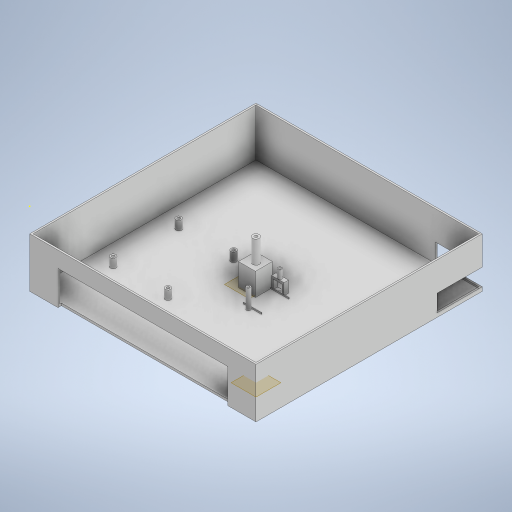
# Autodesk Inventor part: Box
Saved by Autodesk Inventor 2024 (Build 280153000, 153)
## iProperties
Created: 2023-12-20
Part Number: Box
Material: Generic
Document SubType Name: Modeling
Designer: 96279
Density: 1 g/cm^3
Appearance: Default
Author: 96279
Autodesk Inventor part; units mm, degrees
ref_plane "YZ Plane" through (0, 0, 0) normal (1, 0, 0) x (0, 1, 0)
ref_plane "XZ Plane" through (0, 0, 0) normal (0, 1, 0) x (-1, 0, 0)
ref_plane "XY Plane" through (0, 0, 0) normal (0, 0, 1) x (1, 0, 0)
sketch "Sketch1" plane through (0, 0, 0) normal (0, 1, 0) x (-1, 0, 0)
  line L0 (0, 0) -> (200, 0)
  line L1 (200, 0) -> (200, -200)
  line L2 (200, -200) -> (0, -200)
  line L3 (0, -200) -> (0, 0)
  line L4 (198, -198) -> (198, -2)
  line L5 (198, -2) -> (2, -2)
  line L6 (2, -2) -> (2, -198)
  line L7 (2, -198) -> (198, -198)
  dimension "d0" = 200
  dimension "d1" = 200
  dimension "d2" = 2
  constraints: 16 end point, 4 parallel, 2 perpendicular, 1 horizontal, 3 other
  measures "d0" distance of L0.end L1.end
  measures "d1" distance of L1.end L2.end
  measures "d2" distance between parallel lines of L1 L4
extrude "Extrusion1" add sketch "Sketch1" against normal blind 65 contours L0 L1 L2 L3 | L7 L6 L5 L4
sketch "Sketch2" plane through (0, 0, 0) normal (0, 1, 0) x (1, 0, 0)
  line L0 (-198.5, 198.5) -> (-1.5, 198.5)
  line L1 (-1.5, 198.5) -> (-1.5, 1.5)
  line L2 (-1.5, 1.5) -> (-198.5, 1.5)
  line L3 (-198.5, 1.5) -> (-198.5, 198.5)
  line L4 (-200, 200) -> (-200, 0) projected
  line L5 (0, 200) -> (-200, 200) projected
  line L6 (-109.0225, 121.8048) -> (-59.0225, 121.8048)
  line L7 (-59.0225, 121.8048) -> (-59.0225, 76.8048)
  line L8 (-59.0225, 76.8048) -> (-109.0225, 76.8048)
  line L9 (-109.0225, 76.8048) -> (-109.0225, 121.8048)
  circle A0 centre (-100, 100) radius 4
  point P0 (0, 0)
  dimension "d5" = 197
  dimension "d6" = 197
  dimension "d7" = 1.5
  dimension "d8" = 1.5
  dimension "d37" = 50
  dimension "d38" = 45
  dimension "d39" = 8
  constraints: 16 end point, 4 parallel, 2 horizontal, 2 perpendicular, 1 centre point
  measures "d5" distance of L0.end L1.end
  measures "d6" distance of L0.start L0.end
  measures "d7" distance between parallel lines of L3 L4
  measures "d8" distance between parallel lines of L0 L5
  measures "d37" distance of L6.start L6.end
  measures "d38" distance of L6.end L7.end
  measures "d39" diameter of A0
extrude "Extrusion2" cut sketch "Sketch2" against normal blind 63 contours L0 L1 L2 L3 | L6 L7 L8 L9 | A0
sketch "Sketch3" plane through (-200, 0, 0) normal (0, 0, 1) x (1, 0, 0)
  line L0 (25, -35) -> (25, -65)
  line L1 (25, -65) -> (175, -65)
  line L2 (175, -65) -> (175, -35)
  line L3 (175, -35) -> (25, -35)
  line L4 (200, 0) -> (200, -65) projected
  line L5 (42.8625, -63) -> (47.625, -63)
  line L6 (198.5, -63) -> (1.5, -63) projected
  line L7 (200, -65) -> (0, -65) projected
  dimension "d11" = 150
  dimension "d12" = 30
  dimension "d13" = 25
  dimension "d14" = 0
  dimension "d36" = 0
  constraints: 10 end point, 2 parallel, 1 perpendicular
  measures "d11" distance of L2.end L0.start
  measures "d12" distance of L1.end L2.end
  measures "d13" distance between parallel lines of L2 L4
  measures "d14" distance between parallel lines of L5 L6
  measures "d36" distance between parallel lines of L7 L1
extrude "Extrusion3" cut sketch "Sketch3" against normal blind 3
sketch "Sketch4" plane through (0, 0, -200) normal (0, 0, -1) x (-1, 0, 0)
  line L0 (40.0009, -61.5) -> (40.0009, -46.5)
  line L1 (0.0009, -46.5) -> (40.0009, -46.5)
  line L2 (40.0009, -61.5) -> (0.0009, -61.5)
  line L3 (0.0009, -61.5) -> (0.0009, -46.5)
  line L4 (0.0009, -46.5) -> (40.0009, -46.5)
  line L5 (40.0009, -46.5) -> (40.0009, -61.5)
  line L6 (200, -65) -> (0, -65) projected
  point P0 (48.3834, -59.8808)
  point P1 (40.0009, -54)
  point P2 (0.0009, -54)
  dimension "d27" = 40
  dimension "d28" = 15
  dimension "d29" = 3.5
  constraints: 12 end point, 2 midpoint, 2 parallel, 1 horizontal, 1 perpendicular
  measures "d27" distance of L0.start L2.end
  measures "d28" distance of L0.start L0.end
  measures "d29" distance between parallel lines of L6 L2
extrude "Extrusion4" cut sketch "Sketch4" against normal blind 3
sketch "Sketch5" plane through (0, 0, 0) normal (1, 0, 0) x (0, 0, -1)
  line L0 (200, -61.5) -> (160, -61.5)
  line L1 (160, -61.5) -> (160, -46.5)
  line L2 (160, -46.5) -> (200, -46.5)
  line L3 (200, -46.5) -> (200, -61.5)
  point P0 (0, 0)
  point P1 (160, -54)
  dimension "d30" = 40
  dimension "d33" = 15
  constraints: 8 end point, 2 parallel, 1 horizontal, 1 midpoint, 1 perpendicular
  measures "d30" distance of L0.start L0.end
  measures "d33" distance of L0.end L1.end
extrude "Extrusion5" cut sketch "Sketch5" against normal blind 3
ref_plane "Work Plane4" through (-100, -62, -100) normal (0, 1, 0) x (1, 0, 0)
sketch "Sketch7" plane through (-100, -62, -100) normal (0, 1, 0) x (1, 0, 0)
  line L0 (31.2315, 20.7219) -> (-8.7685, 20.7219) projected
  line L1 (-8.7685, -19.2781) -> (31.2315, -19.2781) projected
  line L2 (-8.7685, 20.7219) -> (7.9375, 20.7219)
  line L3 (7.9375, 20.7219) -> (7.9375, -19.2781)
  line L4 (7.9375, -19.2781) -> (-8.7685, -19.2781)
  line L5 (-8.7685, -19.2781) -> (-8.7685, 20.7219)
  circle A0 centre (0, 0) radius 3
  point P0 (100, -100)
  dimension "d51" = 6
  constraints: 8 end point, 2 parallel, 1 centre point, 1 horizontal, 1 perpendicular, 1 point on line
  measures "d51" diameter of A0
extrude "Extrusion7" add sketch "Sketch7" along normal blind 39 contours A0
ref_plane "Work Plane3" through (0, -35, 0) normal (0, 1, 0) x (1, 0, 0)
sketch "Sketch9" plane through (-100, -23, -100) normal (0, 1, 0) x (1, 0, 0)
  point P0 (100, -100)
  point P1 (-0.0134, 0.0104)
hole "Hole1" at (-100.0134, -23, -100.0104) direction (0, -1, 0) diameter 2.7 depth 5
sketch "Sketch16" plane through (0, -63, 0) normal (0, 1, 0) x (1, 0, 0)
  line L0 (-183.7981, 135.019) -> (-127.7981, 135.019)
  line L1 (-127.7981, 135.019) -> (-127.7981, 50.019)
  line L2 (-127.7981, 50.019) -> (-183.7981, 50.019)
  line L3 (-183.7981, 50.019) -> (-183.7981, 135.019)
  circle A0 centre (-131.5481, 111.769) radius 2.5
  circle A1 centre (-131.5481, 53.769) radius 2.5
  circle A2 centre (-180.0481, 111.769) radius 2.5
  circle A3 centre (-180.0481, 53.769) radius 2.5
  point P0 (0, 0)
  dimension "d106" = 85
  dimension "d107" = 56
  dimension "d108" = 5
  dimension "d109" = 5
  dimension "d110" = 23.25
  dimension "d111" = 58
  dimension "d112" = 3.75
  dimension "d113" = 5
  dimension "d114" = 5
  dimension "d115" = 58
  dimension "d116" = 23.25
  dimension "d117" = 48.5
  dimension "d118" = 3.75
  dimension "d119" = 3.75
  dimension "d120" = 48.5
  constraints: 8 end point, 4 centre point, 2 parallel, 1 horizontal, 1 perpendicular
  measures "d106" distance of L0.end L1.end
  measures "d107" distance of L1.end L2.end
  measures "d108" diameter of A0
  measures "d109" diameter of A1
  measures "d110" distance from line of A0.centre L0
  measures "d111" distance of A1.centre A0.centre
  measures "d112" distance from line of L2 A1.centre
  measures "d113" diameter of A3
  measures "d114" diameter of A2
  measures "d115" distance of A3.centre A2.centre
  measures "d116" distance from line of A2.centre L0
  measures "d117" distance of A2.centre A0.centre
  measures "d118" distance from line of A0.centre L1
  measures "d119" distance from line of L1 A1.centre
  measures "d120" distance of A3.centre A1.centre
extrude "Extrusion14" add sketch "Sketch16" along normal blind 8 contours A0 | A1 | A2 | A3
sketch "Sketch18" plane through (-180.0481, -55, -111.769) normal (0, 1, 0) x (1, 0, 0)
  point P0 (180.0481, -111.769)
  point P1 (0.0125, -0.0104)
hole "Hole4" at (-180.0357, -55, -111.7586) direction (0, -1, 0) diameter 2.6 depth 5
sketch "Sketch19" plane through (-131.5481, -55, -111.769) normal (0, 1, 0) x (1, 0, 0)
  point P0 (131.5481, -111.769)
  point P1 (0.007, -0.059)
hole "Hole5" at (-131.5412, -55, -111.7101) direction (0, -1, 0) diameter 2.6 depth 5
sketch "Sketch20" plane through (-180.0481, -55, -53.769) normal (0, 1, 0) x (1, 0, 0)
  point P0 (180.0481, -53.769)
  point P1 (0.0525, -0.0221)
hole "Hole6" at (-179.9956, -55, -53.747) direction (0, -1, 0) diameter 2.6 depth 5
sketch "Sketch21" plane through (-131.5481, -55, -53.769) normal (0, 1, 0) x (1, 0, 0)
  point P0 (131.5481, -53.769)
  point P1 (0.0019, 0.0101)
hole "Hole7" at (-131.5462, -55, -53.7792) direction (0, -1, 0) diameter 2.6 depth 5
sketch "Sketch23" plane through (-200, 0, 0) normal (0, 0, 1) x (1, 0, 0)
  line L0 (200, 0) -> (200, -65) projected
  line L1 (-0.0001, 0) -> (200, 0)
  line L2 (200, 0) -> (200, -21)
  line L3 (200, -21) -> (-0.0001, -21)
  line L4 (-0.0001, -21) -> (-0.0001, 0)
  dimension "d158" = 21
  constraints: 8 end point, 2 parallel, 1 horizontal, 1 perpendicular, 1 point on line
  measures "d158" distance of L3.end L1.start
extrude "Extrusion15" cut sketch "Sketch23" against normal blind 3
sketch "Sketch24" plane through (0, -65, 0) normal (1, 0, 0) x (0, 0, -1)
  line L0 (2.6301, 65) -> (209.4801, 65)
  line L1 (209.4801, 65) -> (209.4801, 44)
  line L2 (209.4801, 44) -> (2.6301, 44)
  line L3 (2.6301, 44) -> (2.6301, 65)
  point P0 (0, 65)
  point P1 (-254.0504, -31.9889)
  dimension "d161" = 21
  constraints: 8 end point, 2 parallel, 1 horizontal, 1 perpendicular
  measures "d161" distance of L2.end L0.start
extrude "Extrusion16" cut sketch "Sketch24" against normal blind 1.5
sketch "Sketch25" plane through (0, -65, -200) normal (0, 0, -1) x (-1, 0, 0)
  line L0 (198.5, 65) -> (1.5, 65) projected
  line L1 (1.5, 65) -> (200, 65)
  line L2 (200, 65) -> (200, 44)
  line L3 (200, 44) -> (1.5, 44)
  line L4 (1.5, 44) -> (1.5, 65)
  point P0 (0, 65)
  dimension "d164" = 21
  constraints: 8 end point, 2 parallel, 1 horizontal, 1 perpendicular
  measures "d164" distance of L1.end L2.end
extrude "Extrusion17" cut sketch "Sketch25" against normal blind 1.5
sketch "Sketch29" plane through (0, -63, 0) normal (0, 1, 0) x (1, 0, 0)
  circle A0 centre (-87.6204, 99.9966) radius 2.4
  circle A1 centre (-100.007, 99.1404) radius 1.5875
  line L0 (-81.6277, 78.5588) -> (-81.6277, 83.3088)
  line L1 (-81.6277, 83.3088) -> (-93.6277, 83.3088)
  line L2 (-93.6277, 83.3088) -> (-93.6277, 78.5588)
  line L3 (-93.6277, 83.3088) -> (-81.6132, 83.3088)
  line L4 (-81.6132, 83.3088) -> (-81.6132, 106.3088)
  line L5 (-81.6132, 106.3088) -> (-93.6277, 106.3088)
  line L6 (-93.6277, 106.3088) -> (-93.6277, 83.3088)
  line L7 (-93.6277, 106.3088) -> (-81.6132, 106.3088)
  line L8 (-81.6132, 106.3088) -> (-81.6132, 111.0588)
  line L9 (-93.6277, 111.0588) -> (-93.6277, 106.3088)
  arc A2 (-87.2339, 79.8817) -> (-88.0214, 79.8817) centre (-87.6277, 80.9088) ccw
  arc A3 (-87.9871, 109.7433) -> (-87.2394, 109.7433) centre (-87.6132, 108.7088) ccw
  line L10 (-88.0214, 79.8817) -> (-88.0068, 79.8817)
  line L11 (-88.0068, 78.5588) -> (-88.0214, 78.5588)
  line L12 (-88.0214, 78.5588) -> (-88.0214, 79.8817)
  line L13 (-88.0214, 79.8817) -> (-88.0068, 79.8817)
  line L14 (-88.0068, 78.5588) -> (-88.0214, 78.5588)
  line L15 (-88.0214, 78.5588) -> (-88.0214, 79.8817)
  line L16 (-148.191, 49.2124) -> (-151.9502, 49.2124)
  line L17 (-87.2339, 79.8817) -> (-87.2339, 78.5588)
  line L18 (-88.0068, 109.7433) -> (-88.0068, 111.0662)
  line L19 (-88.0068, 109.7433) -> (-88.0068, 111.0662)
  line L20 (-87.613, 87.7328) -> (-87.613, 87.7254)
  line L21 (-87.2193, 111.0662) -> (-87.2193, 109.7433)
  line L22 (-87.9871, 109.7433) -> (-88.0068, 109.7433)
  line L23 (-87.9871, 109.7433) -> (-88.0068, 109.7433)
  line L24 (-87.2193, 109.7433) -> (-87.2394, 109.7433)
  line L25 (-87.2339, 111.0662) -> (-87.2193, 111.0662)
  circle A4 centre (-87.6132, 100.0088) radius 2.4
  circle A5 centre (-87.6132, 100.0088) radius 5.7525
  line L26 (-93.6277, 78.5588) -> (-88.0214, 78.5588)
  line L27 (-87.2339, 78.5588) -> (-81.6277, 78.5588)
  line L28 (-81.6132, 111.0588) -> (-87.2193, 111.0588)
  line L29 (-88.0068, 111.0588) -> (-93.6277, 111.0588)
  circle A6 centre (-87.6277, 80.9088) radius 1.75
  circle A7 centre (-87.6132, 108.7088) radius 1.75
  point P0 (0, 0)
  point P1 (-365.9025, -227.0891)
  point P2 (-350.612, -204.1468)
  point P3 (-350.6265, -227.1468)
  point P4 (-145.8741, 48.5842)
  dimension "d178" = 12.3867
  dimension "d186" = 12
  dimension "d187" = 4.75
  dimension "d188" = 23
  dimension "d189" = 4.75
  dimension "d190" = 2.2
  dimension "d191" = 2.2
  dimension "d192" = -27.8
  dimension "d193" = 4.8
  dimension "d196" = 3.5
  dimension "d197" = 3.5
  constraints: 60 end point, 12 parallel, 8 centre point, 5 perpendicular, 5 point on line, 4 point on circle, 3 coincident
  measures "d178" horizontal distance of A0.centre A1.centre
  measures "d186" distance of L0.end L1.end
  measures "d187" distance of L1.end L2.end
  measures "d188" distance of L5.end L1.end
  measures "d189" distance of L9.start L5.end
  measures "d190" diameter of A2
  measures "d191" diameter of A3
  measures "d192" distance of A3.centre A2.centre
  measures "d193" diameter of A4
  measures "d196" diameter of A7
  measures "d197" diameter of A6
sketch "Sketch30" plane through (0, -63, 0) normal (0, 1, 0) x (1, 0, 0)
  line L0 (-108.5304, 108.0352) -> (-93.5304, 108.0352)
  line L1 (-93.5304, 108.0352) -> (-93.5304, 93.0352)
  line L2 (-93.5304, 93.0352) -> (-108.5304, 93.0352)
  line L3 (-108.5304, 93.0352) -> (-108.5304, 108.0352)
  point P0 (0, 0)
  dimension "d171" = 15
  dimension "d172" = 15
  constraints: 8 end point, 2 parallel, 1 horizontal, 1 perpendicular
  measures "d171" distance of L0.start L0.end
  measures "d172" distance of L0.end L1.end
extrude "Extrusion19" add sketch "Sketch30" along normal blind 20
sketch "Sketch31" plane through (-200, -65, -200) normal (-1, 0, 0) x (0, 0, 1)
  point P0 (200, 65)
sketch "Sketch32" plane through (-200, -65, -200) normal (-1, 0, 0) x (0, 0, 1)
  line L0 (1.5, 65) -> (0, 65) projected
  line L1 (0, 65) -> (197, 65)
  line L2 (197, 65) -> (197, 44)
  line L3 (197, 44) -> (0, 44)
  line L4 (0, 44) -> (0, 65)
  point P0 (200, 65)
  constraints: 8 end point, 2 parallel, 1 horizontal, 1 perpendicular
extrude "Extrusion20" cut sketch "Sketch32" against normal blind 1.5
sketch "Sketch34" plane through (0, -63, 0) normal (0, 1, 0) x (1, 0, 0)
  line L0 (-93.5304, 106.9186) -> (-77.5304, 106.9186)
  line L1 (-77.5304, 106.9186) -> (-77.5304, 106.4186)
  line L2 (-77.5304, 106.4186) -> (-93.5304, 106.4186)
  line L3 (-93.5304, 106.4186) -> (-93.5304, 106.9186)
  line L4 (-93.9801, 83.2121) -> (-77.9801, 83.2121)
  line L5 (-77.9801, 83.2121) -> (-77.9801, 82.7121)
  line L6 (-77.9801, 82.7121) -> (-93.9801, 82.7121)
  line L7 (-93.9801, 82.7121) -> (-93.9801, 83.2121)
  point P0 (0, 0)
  dimension "d179" = 16
  dimension "d180" = 0.5
  dimension "d181" = 16
  dimension "d182" = 0.5
  constraints: 16 end point, 4 parallel, 2 horizontal, 2 perpendicular
  measures "d179" distance of L0.start L0.end
  measures "d180" distance of L0.end L1.end
  measures "d181" distance of L4.start L4.end
  measures "d182" distance of L4.end L5.end
extrude "Extrusion21" add sketch "Sketch34" along normal blind 1
extrude "Extrusion22" add sketch "Sketch29" along normal blind 17.3 contours A6 L12 A2 L17 | L17 A2 L12 A6 | A7 L21 L24 A3 L22 L18 | L18 L22 A3 L24 L21 A7
sketch "Sketch35" plane through (-87.6132, -45.7, -108.7088) normal (0, 1, 0) x (1, 0, 0)
  circle A0 centre (0, 0) radius 1
  circle A1 centre (0, -27.804) radius 1
  point P0 (87.6132, -108.7088)
  dimension "d200" = 2
  dimension "d201" = 2
  constraints: 2 centre point
  measures "d200" diameter of A0
  measures "d201" diameter of A1
hole "Hole8" at (-87.6132, -45.7, -108.7088) at (-87.6132, -45.7, -80.9048) direction (0, -1, 0) diameter 2 depth 30
sketch "Sketch36" plane through (0, -63, 0) normal (0, 1, 0) x (1, 0, 0)
  line L0 (-77.5304, 106.9186) -> (-93.5304, 106.9186) projected
  line L1 (-93.2842, 110.9186) -> (-82.1811, 110.9186)
  line L2 (-82.1811, 110.9186) -> (-82.1811, 106.9186)
  line L3 (-82.1811, 106.9186) -> (-93.2842, 106.9186)
  line L4 (-93.2842, 106.9186) -> (-93.2842, 110.9186)
  point P0 (0, 0)
  dimension "d212" = 4
  constraints: 8 end point, 2 parallel, 1 horizontal, 1 perpendicular, 1 point on line
  measures "d212" distance of L1.end L2.end
extrude "Extrusion23" add sketch "Sketch36" along normal blind 10
sketch "Sketch37" plane through (-82.1811, -63, -110.9186) normal (0, 0, -1) x (-1, 0, 0)
  line L0 (1.5875, 8.0595) -> (9.525, 8.0595)
  line L1 (9.525, 8.0595) -> (9.525, 0.0595)
  line L2 (9.525, 0.0595) -> (1.5875, 0.0595)
  line L3 (1.5875, 0.0595) -> (1.5875, 8.0595)
  point P0 (-82.1811, 63)
  dimension "d211" = 8
  constraints: 8 end point, 2 parallel, 1 horizontal, 1 perpendicular
  measures "d211" distance of L0.end L1.end
extrude "Extrusion24" cut sketch "Sketch37" against normal blind 4
body "Solid1"
